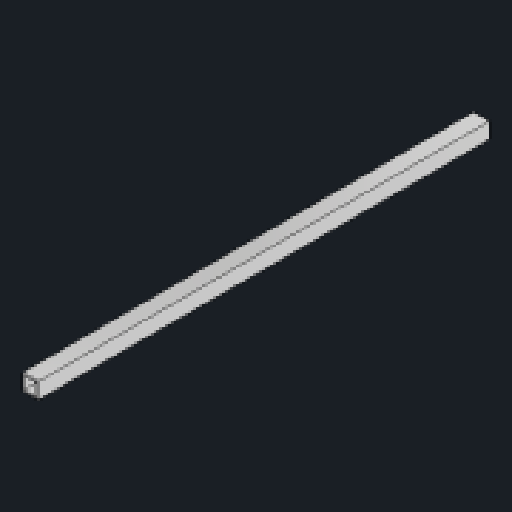
# Autodesk Inventor part: Rail
Saved by Autodesk Inventor 2023.2 (Build 272271030, 271C)
## iProperties
Created: 2024-02-19
Part Number: Rail
Material: Aluminum 6061
Document SubType Name: Modeling
Designer: robpl
Density: 2.7 g/cm^3
Appearance: Aluminum - Dark
Mass: 1.1988 g
Surface Area: 22.2888 cm^2
Volume: 0.444 cm^3
Author: robpl
Autodesk Inventor part; units mm, degrees
ref_plane "YZ Plane" through (0, 0, 0) normal (1, 0, 0) x (0, 1, 0)
ref_plane "XZ Plane" through (0, 0, 0) normal (0, 1, 0) x (-1, 0, 0)
ref_plane "XY Plane" through (0, 0, 0) normal (0, 0, 1) x (1, 0, 0)
sketch "Sketch1" plane through (0, 0, 0) normal (0, 0, 1) x (1, 0, 0)
  line L0 (-1.5875, 1.5875) -> (1.5875, 1.5875)
  line L1 (1.5875, 1.5875) -> (1.5875, -1.5875)
  line L2 (1.5875, -1.5875) -> (-1.5875, -1.5875)
  line L3 (-1.5875, -1.5875) -> (-1.5875, 1.5875)
  line L4 (-1.5875, 1.5875) -> (1.5875, -1.5875) construction
  line L5 (1.5875, 1.5875) -> (-1.5875, -1.5875) construction
  line L6 (-1.1875, -1.1875) -> (1.1875, -1.1875)
  line L7 (1.1875, -1.1875) -> (1.1875, 1.1875)
  line L8 (1.1875, 1.1875) -> (-1.1875, 1.1875)
  line L9 (-1.1875, 1.1875) -> (-1.1875, -1.1875)
  point P0 (0, 0)
  dimension "d0" = 3.175
  dimension "d1" = 0.4
  constraints: 20 end point, 4 parallel, 3 perpendicular, 2 midpoint, 1 horizontal, 3 other
  measures "d0" distance of L2.end L0.start
  measures "d1" distance between parallel lines of L2 L6
extrude "Extrusion1" add sketch "Sketch1" along normal blind 90
body "Solid1"
